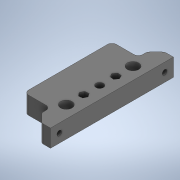
# Autodesk Inventor part: Stationaryjaw2
Saved by Autodesk Inventor 2020.2 (Build 242310000, 310)
## iProperties
Created: 2021-06-22
Part Number: Stationaryjaw2
Material: Generic
Document SubType Name: Modeling
Designer: JK
Density: 1 g/cm^3
Appearance: Gray
Author: JK
Autodesk Inventor part; units mm, degrees
ref_plane "YZ Plane" through (0, 0, 0) normal (1, 0, 0) x (0, 1, 0)
ref_plane "XZ Plane" through (0, 0, 0) normal (0, 1, 0) x (-1, 0, 0)
ref_plane "XY Plane" through (0, 0, 0) normal (0, 0, 1) x (1, 0, 0)
sketch "Sketch1" plane through (0, 0, 0) normal (0, 1, 0) x (-1, 0, 0)
  line L0 (-25, 50) -> (25, 50)
  line L1 (25, 50) -> (25, -50)
  line L2 (25, -50) -> (-25, -50)
  line L3 (-25, -50) -> (-25, 50)
  line L4 (-25, 50) -> (25, -50) construction
  line L5 (25, 50) -> (-25, -50) construction
  circle A0 centre (-11, 38) radius 6.5
  circle A1 centre (-11, -38) radius 6.5
  point P0 (0, 0)
  dimension "d0" = 13
  dimension "d1" = 13
  dimension "d2" = 100
  dimension "d3" = 50
  dimension "d4" = 12
  dimension "d6" = 14
  dimension "d7" = 12
  constraints: 12 end point, 2 centre point, 2 midpoint, 2 parallel, 1 horizontal, 1 perpendicular, 1 vertical alignment
  measures "d0" diameter of A0
  measures "d1" diameter of A1
  measures "d2" distance of L0.end L1.end
  measures "d3" distance of L1.end L2.end
  measures "d4" distance from line of L0 A0.centre
  measures "d6" distance from line of L3 A1.centre
  measures "d7" distance from line of L2 A1.centre
extrude "Extrusion1" add sketch "Sketch1" along normal blind 20
sketch "Sketch2" plane through (0, 0, 0) normal (0, -1, 0) x (1, 0, 0)
  circle A0 centre (11, -38) radius 6.5 projected
  circle A1 centre (11, -38) radius 4
  circle A2 centre (11, 38) radius 6.5 projected
  circle A3 centre (11, 38) radius 4
  point P0 (0, 0)
  dimension "d10" = 8
  dimension "d11" = 8
  constraints: 2 centre point, 2 coincident
  measures "d10" diameter of A1
  measures "d11" diameter of A3
extrude "Extrusion2" add sketch "Sketch2" against normal blind 5
fillet "Fillet1" radius 5 2 edges at (-25, 10, -50) (-25, 10, 50)
sketch "Sketch3" plane through (0, 0, 0) normal (0, -1, 0) x (1, 0, 0)
  circle A0 centre (11, 0) radius 4.25
  circle A1 centre (11, -38) radius 4 projected
  circle A2 centre (11, -18.25) radius 2.65
  circle A3 centre (11, 18.25) radius 2.65
  point P0 (0, 0)
  dimension "d15" = 8.5
  dimension "d16" = 5.3
  dimension "d17" = 18.25
  dimension "d18" = 18.25
  constraints: 3 centre point, 1 equal radius, 1 vertical alignment
  measures "d15" diameter of A0
  measures "d16" diameter of A2
  measures "d17" distance of A0.centre A2.centre
  measures "d18" distance of A0.centre A3.centre
extrude "Extrusion3" cut sketch "Sketch3" against normal through all contours A0 | A2 | A3
sketch "Sketch4" plane through (0, 20, 0) normal (0, 1, 0) x (1, 0, 0)
  circle A0 centre (11, -18.25) radius 2.65 projected
  circle A1 centre (11, -18.25) radius 4.1
  circle A2 centre (11, 18.25) radius 2.65 projected
  circle A3 centre (11, 18.25) radius 4.1
  line L0 (6.2846, -18.672) -> (8.2769, -14.3773)
  line L1 (8.2769, -14.3773) -> (12.9923, -13.9553)
  line L2 (12.9923, -13.9553) -> (15.7154, -17.828)
  line L3 (15.7154, -17.828) -> (13.7231, -22.1227)
  line L4 (13.7231, -22.1227) -> (9.0077, -22.5447)
  line L5 (9.0077, -22.5447) -> (6.2846, -18.672)
  line L6 (6.2821, 18.6431) -> (8.9814, 22.5324)
  line L7 (8.9814, 22.5324) -> (13.6994, 22.1393)
  line L8 (13.6994, 22.1393) -> (15.7179, 17.8569)
  line L9 (15.7179, 17.8569) -> (13.0186, 13.9676)
  line L10 (13.0186, 13.9676) -> (8.3006, 14.3607)
  line L11 (8.3006, 14.3607) -> (6.2821, 18.6431)
  point P0 (0, 0)
  dimension "d21" = 8.2
  constraints: 24 end point, 4 coincident, 2 centre point, 2 tangent, 1 equal radius, 26 other
  measures "d21" diameter of A1
extrude "Extrusion4" cut sketch "Sketch4" against normal blind 8 contours A0 | A1 | A1 L2 L3 | A1 L1 L2 | L3 L4 A1 | A1 L0 L1 | L4 L5 A1 | A1 L5 L0 | A2 | A3 | A3 L8 L9 | A3 L7 L8 | L9 L10 A3 | A3 L6 L7 | L10 L11 A3 | A3 L11 L6
sketch "Sketch6" plane through (25, 0, 50) normal (1, 0, 0) x (0, 0, -1)
  line L0 (0, 20) -> (-20, 20)
  line L1 (-20, 20) -> (-20, 0)
  line L2 (-20, 0) -> (0, 0)
  line L3 (0, 0) -> (0, 20)
  line L4 (100, 0) -> (100, 20) projected
  line L5 (100, 20) -> (120, 20)
  line L6 (120, 20) -> (120, 0)
  line L7 (120, 0) -> (100, 0)
  line L8 (100, 0) -> (100, 20)
  line L9 (0, 0) -> (0, 20) projected
  circle A0 centre (-10, 10) radius 2.75
  circle A1 centre (110, 10) radius 2.75
  point P0 (50, 0)
  dimension "d26" = 20
  dimension "d27" = 20
  dimension "d28" = 20
  dimension "d29" = 5.5
  constraints: 16 end point, 4 parallel, 2 centre point, 2 collinear, 2 horizontal, 2 perpendicular, 1 equal radius, 1 point on line
  measures "d26" distance between parallel lines of L1 L3
  measures "d27" distance between parallel lines of L5 L7
  measures "d28" distance between parallel lines of L4 L6
  measures "d29" diameter of A0
extrude "Extrusion5" add sketch "Sketch6" against normal blind 20
chamfer "Chamfer1" distance 10 angle 45 2 edges at (5, 10, 70) (5, 10, -70)
sketch "Sketch7" plane through (5, 0, 50) normal (-1, 0, 0) x (0, 0, 1)
  circle A0 centre (10, 10) radius 2.75 projected
  circle A1 centre (10, 10) radius 4.75
  arc A2 (-110, 12.75) -> (-110, 7.25) centre (-110, 10) ccw projected
  circle A3 centre (-110, 10) radius 4.75
  point P0 (-50, 0)
  dimension "d35" = 9.5
  constraints: 2 centre point, 2 coincident, 1 equal radius
  measures "d35" diameter of A1
extrude "Extrusion6" cut sketch "Sketch7" against normal blind 10 contours A0 | A1 | A3
fillet "Fillet2" radius 5 8 edges at (5, 10, -50) (5, 17.375, -60) (5, 2.625, -60) (15, 10, -70) (5, 2.625, 60) (5, 17.375, 60) (5, 10, 50) (15, 10, 70)
body "Solid1"
